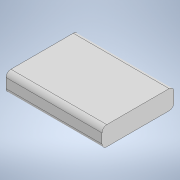
# Autodesk Inventor part: lipol-70mAh
Saved by Autodesk Inventor 2022.3 (Build 263350000, 350)
## iProperties
Created: 2022-12-14
Part Number: lipol-70mAh
Material: Generic
Document SubType Name: Modeling
Designer: komputer
Density: 1 g/cm^3
Appearance: Default
Author: komputer
Autodesk Inventor part; units mm, degrees
ref_plane "YZ Plane" through (0, 0, 0) normal (1, 0, 0) x (0, 1, 0)
ref_plane "XZ Plane" through (0, 0, 0) normal (0, 1, 0) x (-1, 0, 0)
ref_plane "XY Plane" through (0, 0, 0) normal (0, 0, 1) x (1, 0, 0)
sketch "Sketch1" plane through (0, 0, 0) normal (0, 1, 0) x (-1, 0, 0)
  line L0 (3.5859, 5.0732) -> (-16.4141, 5.0732)
  line L1 (-16.4141, 5.0732) -> (-16.4141, -9.9268)
  line L2 (-16.4141, -9.9268) -> (3.5859, -9.9268)
  line L3 (3.5859, -9.9268) -> (3.5859, 5.0732)
  point P0 (0, 0)
  dimension "d0" = 20
  dimension "d1" = 15
  constraints: 8 end point, 2 parallel, 1 horizontal, 1 perpendicular
  measures "d0" distance of L2.end L1.end
  measures "d1" distance of L1.end L0.end
extrude "Extrusion1" add sketch "Sketch1" along normal blind 4
fillet "Fillet1" radius 1 4 edges at (6.4141, 4, -9.9268) (6.4141, 4, 5.0732) (6.4141, 0, 5.0732) (6.4141, 0, -9.9268)
body "Solid1"
